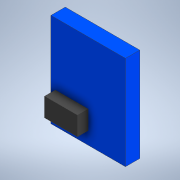
# Autodesk Inventor part: tof
Saved by Autodesk Inventor 2022.3 (Build 263350000, 350)
## iProperties
Created: 2022-12-13
Part Number: tof
Material: Generic
Document SubType Name: Modeling
Designer: komputer
Density: 1 g/cm^3
Appearance: Default
Author: komputer
Autodesk Inventor part; units mm, degrees
ref_plane "YZ Plane" through (0, 0, 0) normal (1, 0, 0) x (0, 1, 0)
ref_plane "XZ Plane" through (0, 0, 0) normal (0, 1, 0) x (-1, 0, 0)
ref_plane "XY Plane" through (0, 0, 0) normal (0, 0, 1) x (1, 0, 0)
sketch "Sketch1" plane through (0, 0, 0) normal (0, 0, 1) x (1, 0, 0)
  line L0 (-4.1767, 5.9085) -> (6.2233, 5.9085)
  line L1 (6.2233, 5.9085) -> (6.2233, -7.1915)
  line L2 (6.2233, -7.1915) -> (-4.1767, -7.1915)
  line L3 (-4.1767, -7.1915) -> (-4.1767, 5.9085)
  point P0 (0, 0)
  dimension "d0" = 10.4
  dimension "d1" = 13.1
  constraints: 8 end point, 2 parallel, 1 horizontal, 1 perpendicular
  measures "d0" distance of L1.end L2.end
  measures "d1" distance of L0.end L1.end
extrude "Extrusion1" add sketch "Sketch1" along normal blind 2
sketch "Sketch2" plane through (0, 0, 2) normal (0, 0, 1) x (1, 0, 0)
  line L0 (-4.1767, -7.1915) -> (6.2233, -7.1915) projected
  line L1 (6.2233, -7.1915) -> (6.2233, 5.9085) projected
  line L2 (6.2233, 5.9085) -> (-4.1767, 5.9085) projected
  line L3 (-4.1767, 5.9085) -> (-4.1767, -7.1915) projected
  line L4 (6.2233, 5.9085) -> (-4.1767, 5.9085) projected
  line L5 (1.0233, 5.9085) -> (1.0233, -7.1915)
  line L6 (-4.1767, -7.1915) -> (6.2233, -7.1915) projected
  line L7 (6.2233, -7.1915) -> (6.2233, 5.9085) projected
  line L8 (6.2233, -0.6415) -> (-4.1767, -0.6415)
  line L9 (-4.1767, 5.9085) -> (-4.1767, -7.1915) projected
  line L10 (1.0233, -5.4195) -> (-3.5655, -5.4195)
  line L11 (-3.5655, -5.4195) -> (-3.5655, -2.8116)
  line L12 (-3.5655, -2.8116) -> (1.0233, -2.8116)
  line L13 (1.0233, -2.8116) -> (1.0233, -5.4195)
  point P0 (0, 0)
  constraints: 12 end point, 4 midpoint, 2 parallel, 1 horizontal, 1 perpendicular, 1 point on line
extrude "Extrusion2" add sketch "Sketch2" along normal blind 1.5 contours L10 L11 L12 L5
body "Solid1"
